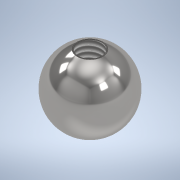
# Autodesk Inventor part: 10mm M4 Ball
Saved by Autodesk Inventor 2022 (Build 260153000, 153)
## iProperties
Created: 2022-03-18
Part Number: 10mm M4 Ball
Material: Generic
Document SubType Name: Modeling
Designer: Nick
Density: 1 g/cm^3
Appearance: Steel - Polished
Author: Nick
Autodesk Inventor part; units mm, degrees
ref_plane "YZ Plane" through (0, 0, 0) normal (1, 0, 0) x (0, 1, 0)
ref_plane "XZ Plane" through (0, 0, 0) normal (0, 1, 0) x (-1, 0, 0)
sketch "Sketch1" plane through (0, 0, 0) normal (0, 0, 1) x (1, 0, 0)
  circle A0 centre (0, 0) radius 5
  line L0 (-1.75, 4.6837) -> (1.75, 4.6837)
  line L1 (0, 6.3391) -> (0, -8.1264)
  point P0 (0, 4.6837)
  point P1 (0, -5)
  dimension "d0" = 10
  dimension "d10" = 3.5
  constraints: 4 end point, 2 point on circle, 1 centre point, 1 coincident, 1 horizontal, 1 vertical, 1 vertical alignment
  measures "d0" diameter of A0
  measures "d10" distance of L0.start L0.end
revolve "Revolution1" add sketch "Sketch1" angle 360 about axis through (0, 6.3391, 0) along (0, -1, 0) picked at (0.3709, -1.7303) contours A0 L1 L0
sketch "Sketch2" plane through (0, 4.6837, 0) normal (0, 1, 0) x (1, 0, 0)
  point P0 (0, 0)
  point P1 (0, 0)
  constraints: 1 coincident
hole "Hole1" at (0, 4.6837, 0) direction (0, -1, 0) diameter 3.242 depth 5 thread size "M4x0.7" class "6H" standard "ANSI Metric M Profile"
ref_plane "Work Plane1" through (0, 4.6837, 0) normal (0, 1, 0) x (1, 0, 0)
body "Solid1"
